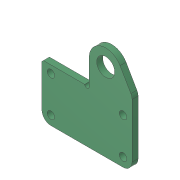
# Autodesk Inventor part: COXA_YAW_SERVO_BASE
Saved by Autodesk Inventor 2019.4 (Build 234330000, 330)
## iProperties
Created: 2019-10-21
Part Number: COXA_YAW_SERVO_BASE
Material: 一般
Document SubType Name: Modeling
Designer: y6tada
Density: 1 g/cm^3
Appearance: 滑らか - 濃い海緑
Author: y6tada
Autodesk Inventor part; units mm, degrees
ref_plane "YZ Plane" through (0, 0, 0) normal (1, 0, 0) x (0, 1, 0)
ref_plane "XZ Plane" through (0, 0, 0) normal (0, 1, 0) x (-1, 0, 0)
ref_plane "XY Plane" through (0, 0, 0) normal (0, 0, 1) x (1, 0, 0)
sketch "スケッチ1" plane through (0, 0, 0) normal (0, 0, 1) x (1, 0, 0)
  line L0 (54.882, 0) -> (12, 60) construction
  line L1 (54.882, 0) -> (70, -21.1529)
  line L2 (70, -21.1529) -> (35, -33.1249)
  line L3 (0, 0) -> (0, 100.7114)
  line L4 (0, 0) -> (54.882, 0) construction
  arc A0 (24.927, 26.5822) -> (24.2651, 18.1082) centre (58.2269, 19.7183) ccw construction
  arc A1 (17.0917, 28.1972) -> (16.274, 17.7294) centre (58.2269, 19.7183) ccw construction
  arc A2 (16.274, 17.7294) -> (24.2651, 18.1082) centre (20.2695, 17.9188) ccw construction
  line L5 (20.2695, 17.9188) -> (58.2269, 19.7183) construction
  line L6 (58.2269, 19.7183) -> (20.6135, 25.1248)
  arc A3 (20.6135, 25.1248) -> (20.2695, 17.9188) centre (58.2269, 19.7183) ccw construction
  line L7 (20.2695, 17.9188) -> (68.8874, -17.2423) construction
  line L8 (68.8874, -17.2423) -> (71.9395, 19.6224) construction
  line L9 (20.6135, 25.1248) -> (35, -33.1249)
  line L10 (20.6135, 25.1248) -> (12, 60) construction
  line L11 (20.6135, 25.1248) -> (54.882, 0) construction
  arc A4 (57.1481, -25.9011) -> (71.9395, 19.6224) centre (54.882, 0) ccw
  line L12 (35, -33.1249) -> (70, -33.1249) construction
  line L13 (70, -33.1249) -> (70, -21.1529) construction
  line L14 (27.4112, -33.1249) -> (45, -293.1249) construction
  line L15 (54.882, 0) -> (53.4072, -2.6124)
  line L16 (54.882, 0) -> (52.2839, -1.5) construction
  arc A5 (52.2839, -1.5) -> (57.7658, -0.8269) centre (54.882, 0) ccw construction
  line L17 (54.882, 0) -> (52.8265, -2.1851) construction
  line L18 (54.882, 0) -> (53.5434, -2.6848) construction
  line L19 (54.882, 0) -> (54.374, -2.9567) construction
  line L20 (54.882, 0) -> (55.2476, -2.9776) construction
  line L21 (54.882, 0) -> (56.0902, -2.7459) construction
  line L22 (54.882, 0) -> (56.8303, -2.2812) construction
  line L23 (54.882, 0) -> (57.4051, -1.6229) construction
  line L24 (54.882, 0) -> (57.7658, -0.8269) construction
  line L25 (58.2269, 19.7183) -> (53.4072, -2.6124)
  line L26 (52.2839, -1.5) -> (58.2269, 19.7183) construction
  line L27 (58.2269, 19.7183) -> (57.7658, -0.8269) construction
  line L28 (55.5792, -7.9696) -> (57.1481, -25.9011) construction
  line L29 (57.8465, -7.4305) -> (64.5165, -24.149) construction
  line L30 (59.8621, -6.2609) -> (71.0674, -20.3478) construction
  line L31 (61.4552, -4.56) -> (76.2448, -14.8199) construction
  line L32 (62.4905, -2.4721) -> (79.6095, -8.0344) construction
  line L33 (62.8801, -0.1745) -> (80.8758, -0.5672) construction
  line L34 (62.591, 2.1379) -> (79.9364, 6.9482) construction
  line L35 (61.6478, 4.2689) -> (76.8709, 13.874) construction
  line L36 (60.1305, 6.0377) -> (71.9395, 19.6224) construction
  arc A6 (55.5792, -7.9696) -> (60.1305, 6.0377) centre (54.882, 0) ccw construction
  line L37 (21.0093, 27.3897) -> (58.2269, 19.7183) construction
  arc A7 (21.0093, 27.3897) -> (20.6135, 25.1248) centre (58.2269, 19.7183) ccw construction
  arc A8 (24.927, 26.5822) -> (17.0917, 28.1972) centre (21.0093, 27.3897) ccw construction
  line L38 (52.8265, -2.1851) -> (58.2269, 19.7183) construction
  line L39 (58.2269, 19.7183) -> (20.7871, 26.2192) construction
  line L40 (20.5792, 24.8807) -> (58.2269, 19.7183) construction
  line L41 (53.5434, -2.6848) -> (58.2269, 19.7183) construction
  line L42 (21.0093, 27.3897) -> (20.7706, -32.6098) construction
  line L43 (20.7706, -32.6098) -> (57.1481, -25.9011) construction
  line L44 (20.7871, 26.2192) -> (28.6655, -33.2613) construction
  line L45 (28.6655, -33.2613) -> (64.5165, -24.149) construction
  line L46 (35, -33.1249) -> (45, -293.1249)
  line L47 (70, -21.1529) -> (45, -293.1249)
  line L48 (28.6655, -33.2613) -> (17.6783, -293.2214) construction
  line L49 (17.6783, -293.2214) -> (64.5165, -24.149) construction
  line L50 (57.1481, -25.9011) -> (-7.4742, -291.2645) construction
  line L51 (-7.4742, -291.2645) -> (20.7706, -32.6098) construction
  line L52 (58.2269, 19.7183) -> (20.4111, 23.4553) construction
  line L53 (58.2269, 19.7183) -> (20.2969, 22.0239) construction
  line L54 (58.2269, 19.7183) -> (20.2388, 20.6688) construction
  line L55 (58.2269, 19.7183) -> (20.2277, 19.4745) construction
  line L56 (58.2269, 19.7183) -> (20.2456, 18.5281) construction
  line L57 (58.2269, 19.7183) -> (54.374, -2.9567) construction
  line L58 (58.2269, 19.7183) -> (55.2476, -2.9776) construction
  line L59 (58.2269, 19.7183) -> (56.0902, -2.7459) construction
  line L60 (58.2269, 19.7183) -> (56.8303, -2.2812) construction
  line L61 (58.2269, 19.7183) -> (57.4051, -1.6229) construction
  line L62 (20.5792, 24.8807) -> (36.3145, -33.0192) construction
  line L63 (36.3145, -33.0192) -> (71.0674, -20.3478) construction
  line L64 (76.2448, -14.8199) -> (43.4556, -31.9429) construction
  line L65 (43.4556, -31.9429) -> (20.4111, 23.4553) construction
  line L66 (20.2969, 22.0239) -> (49.9482, -30.1374) construction
  line L67 (49.9482, -30.1374) -> (79.6095, -8.0344) construction
  line L68 (80.8758, -0.5672) -> (55.7371, -27.7034) construction
  line L69 (55.7371, -27.7034) -> (20.2388, 20.6688) construction
  line L70 (20.2277, 19.4745) -> (60.8132, -24.7162) construction
  line L71 (60.8132, -24.7162) -> (79.9364, 6.9482) construction
  line L72 (76.8709, 13.874) -> (65.1878, -21.2235) construction
  line L73 (65.1878, -21.2235) -> (20.2456, 18.5281) construction
  line L74 (36.3145, -33.0192) -> (51.5259, -292.7664) construction
  line L75 (71.9395, 19.6224) -> (311.1178, -112.2394) construction
  line L76 (311.1178, -112.2394) -> (68.8874, -17.2423) construction
  line L77 (76.8709, 13.874) -> (278.0839, -170.8071) construction
  line L78 (278.0839, -170.8071) -> (65.1878, -21.2235) construction
  line L79 (60.8132, -24.7162) -> (235.5555, -217.4988) construction
  line L80 (235.5555, -217.4988) -> (79.9364, 6.9482) construction
  line L81 (80.8758, -0.5672) -> (187.8232, -251.8758) construction
  line L82 (187.8232, -251.8758) -> (55.7371, -27.7034) construction
  line L83 (49.9482, -30.1374) -> (138.9893, -274.6199) construction
  line L84 (138.9893, -274.6199) -> (79.6095, -8.0344) construction
  line L85 (76.2448, -14.8199) -> (92.626, -287.4468) construction
  line L86 (92.626, -287.4468) -> (43.4556, -31.9429) construction
  line L87 (51.5259, -292.7664) -> (71.0674, -20.3478) construction
  spline S0 degree 4 poles (-7.4742, -291.2645) (-12.2705, -294.3182) (60.154, -292.0463) (27.8526, -295.3281) (110.0905, -286.5066) (139.1565, -274.7713) (216.3886, -242.7571) (259.5293, -197.6399) (297.4502, -150.2821) (311.1178, -112.2394) knots 0 0 0 0 0 0.20634 0.298589 0.40005 0.523805 0.654143 1 1 1 1 1 construction
  spline S1 degree 4 poles (20.7706, -32.6098) (25.5837, -33.2782) (32.3307, -33.6056) (40.6453, -32.8812) (49.7904, -30.3738) (57.6947, -27.0887) (63.1804, -23.3839) (66.7313, -19.9462) (68.8874, -17.2423) knots 0 0 0 0 0 0.335801 0.464563 0.589185 0.709887 1 1 1 1 1
  circle A9 centre (58.2269, 19.7183) radius 4 construction
  line L88 (0, 0) -> (0, -360.4465)
  point P0 (54.882, 0)
  point P1 (54.882, 0)
  point P2 (54.882, 0)
  point P3 (54.882, 0)
  point P4 (54.882, 0)
  point P5 (54.882, 0)
  point P6 (54.882, 0)
  point P7 (54.882, 0)
  dimension "d5" = 60
  dimension "d66" = 26
  dimension "d67" = 35
  dimension "d74" = 65
  dimension "d76" = 3
  dimension "d80" = 134
  dimension "d82" = 20
  dimension "d85" = 134
  dimension "d87" = 65
  dimension "d88" = 60
  dimension "d89" = 86
  dimension "d90" = 86
  dimension "d91" = 86
  dimension "d92" = 4
  dimension "d93" = 86
  dimension "d94" = 86
  dimension "d95" = 95
  dimension "d96" = 86
  dimension "d97" = 86
  dimension "d98" = 86
  dimension "d99" = 86
  dimension "d100" = 86
  dimension "d101" = 8
  dimension "d102" = 12
  dimension "d104" = 74.818
  dimension "d105" = 8
  dimension "d106" = 75.286
  dimension "d111" = 11.972
  dimension "d113" = 70
  dimension "d114" = 38
  dimension "d116" = 90
  dimension "d117" = 260
  constraints: 178 end point, 36 equal length, 28 point on circle, 17 coincident, 14 point on line, 10 centre point, 4 tangent, 2 horizontal, 2 vertical, 1 collinear, 1 concentric, 1 perpendicular, 76 other
  measures "d5" distance from line of L4 L0.end
  measures "d66" radius of A4
  measures "d67" distance of L2.end L12.end
  measures "d74" angle of L15 L1
  measures "d76" radius of A5
  measures "d82" distance of L0.start L5.end
  measures "d87" angle of L16 L28
  measures "d88" distance of L6.end L2.end
  measures "d89" angle of L25 L6
  measures "d90" angle of L26 L37
  measures "d91" angle of L27 L5
  measures "d92" radius of A8
  measures "d93" angle of L38 L39
  measures "d94" angle of L40 L41
  measures "d95" angle of L28 L4
  measures "d96" angle of L57 L52
  measures "d97" angle of L58 L53
  measures "d98" angle of L59 L54
  measures "d99" angle of L55 L60
  measures "d100" angle of L61 L56
  measures "d101" radius of A6
  measures "d102" distance from line of L0.end L3
  measures "d104" angle of L76 L51
  measures "d105" diameter of A9
  measures "d106" angle of L27 L24
  measures "d111" distance of L12.end L1.end
  measures "d113" diameter of L2.end L88
  measures "d114" distance of L5.end L6.end
  measures "d116" diameter of L14.end L88
  measures "d117" distance from line of L14.end L12
sketch "スケッチ2" plane through (0, 0, 0) normal (0, 0, 1) x (1, 0, 0)
  arc A0 (62.99, 22.4683) -> (52.7269, 19.7183) centre (58.2269, 19.7183) ccw
  line L0 (40, 8.7) -> (64, 8.7) construction
  line L1 (64, 8.7) -> (64, -3.3) construction
  line L2 (64, -3.3) -> (40, -3.3) construction
  line L3 (40, -3.3) -> (40, 8.7) construction
  line L4 (36, 10.1673) -> (36, -48.9437) construction
  line L5 (67, 14.719) -> (67, -3.3)
  line L6 (64, -6.3) -> (40, -6.3)
  line L7 (37, -3.3) -> (37, 10.7)
  arc A1 (37, -3.3) -> (40, -6.3) centre (40, -3.3) ccw
  arc A2 (64, -6.3) -> (67, -3.3) centre (64, -3.3) ccw
  line L8 (0, 0) -> (0, -59.5537) construction
  line L9 (10.6628, 2.7) -> (66.9205, 2.7) construction
  line L10 (66.5981, 16.219) -> (62.99, 22.4683)
  arc A3 (67, 14.719) -> (66.5981, 16.219) centre (64, 14.719) ccw
  line L11 (37.5, 11.2) -> (51.2269, 11.2)
  line L12 (52.7269, 19.7183) -> (52.7269, 11.2)
  arc A4 (51.2269, 11.2) -> (52.7269, 11.2) centre (51.9769, 11.2) ccw
  line L13 (37, 10.7) -> (37.5, 11.2)
  point P0 (67, 15.5229)
  point P1 (36.9922, 11.2)
  point P2 (37, 11.2)
  dimension "d16" = 24
  dimension "d17" = 4
  dimension "d18" = 12
  dimension "d20" = 72
  dimension "d23" = 5.5
  dimension "d108" = 3
  dimension "d109" = 30
  dimension "d118" = 2.7
  dimension "d119" = 3
  dimension "d120" = 0.75
  dimension "d121" = 0.5
  dimension "d122" = 0.5
  dimension "d124" = 8.5
  constraints: 28 end point, 10 point on circle, 9 tangent, 6 point on line, 5 centre point, 4 coincident, 4 horizontal, 4 vertical, 3 parallel, 1 perpendicular, 1 other
  measures "d16" distance of L1.end L2.end
  measures "d17" distance between parallel lines of L3 L4
  measures "d18" distance of L2.end L0.start
  measures "d20" diameter of L4 L8
  measures "d23" radius of A0
  measures "d108" radius of A3
  measures "d109" angle of L5 L10
  measures "d118" distance from line of L9 L8.start
  measures "d119" radius of A2
  measures "d120" radius of A4
  measures "d121" distance of L7.end point (37, 11.2)
  measures "d122" distance of L11.start point (37, 11.2)
  measures "d124" distance between parallel lines of L9 L11
extrude "押し出し1" add sketch "スケッチ2" along normal blind 2
hole "穴1" at (58.2269, 19.7183, 0) direction (0, 0, 1) diameter 6 end through all
hole "穴2" at (64, 8.7, 0) at (40, 8.7, 0) at (40, -3.3, 0) at (64, -3.3, 0) direction (0, 0, 1) diameter 2.5 end through all
equation "\"input_link_length\" = 26"
equation "\"input_link_formed_angle\" = 65deg"
equation "\"support_formed_angle\" = 86deg"
equation "\"input_slider_radius\" = 3"
equation "\"driver_rotation_range\" = 134deg"
equation "\"virtual_mass_point_x\" = 12"
equation "\"driver_min_angle\" = 95deg"
equation "\"coupler_x\" = 35"
equation "\"support_link_length\" = 38"
